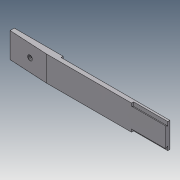
# Autodesk Inventor part: J007777 IMEC DOVE TAIL EXTENSION Rev -
Saved by Autodesk Inventor 2018.3 (Build 223284000, 284)
## iProperties
Created: 2017-01-23
Material: ALUMINUM, 6061-T651
Vendor: HHMI: JRC - ID&F
Document SubType Name: Modeling
Designer: ARNOLDJ
Density: 2.7 g/cm^3
Appearance: Metal-AL-6061 (Machined)
Description: IMEC DOVE TAIL EXTENSION
Project: COMMON
Part Number: J007777 IMEC DOVE TAIL EXTENSION Rev -
RuleStatus: InUse
AfterDocSave0: file://Part Number Cleaner
LAB/DEPT: APIG (SHARED RESOURCE)
REQUESTING SCIENTIST: BARBARTIS, BRIAN
SURFACE ROUGHNESS: 32 Ra
DESIGN DEPARTMENT: HHMI: JRC - ID&F
SPECIAL FINISH: NONE
ALTERED ITEM PART NUMBER: N/A
ALTERED ITEM VENDOR: N/A
ALTERED ITEM DESCRIPTION: N/A
Author: ARNOLDJ
Revision Number: 0
Autodesk Inventor part; units mm, degrees
ref_plane "YZ Plane" through (0, 0, 0) normal (1, 0, 0) x (0, 1, 0)
ref_plane "XZ Plane" through (0, 0, 0) normal (0, 1, 0) x (-1, 0, 0)
ref_plane "XY Plane" through (0, 0, 0) normal (0, 0, 1) x (1, 0, 0)
sketch "Sketch1" plane through (0, 0, 0) normal (0, 0, 1) x (1, 0, 0)
  line L0 (0, 4.2672) -> (0, -4.2672) projected
  line L1 (-26.67, 0) -> (26.67, 0) projected
  line L2 (19.05, -3.048) -> (-19.05, -3.048)
  line L3 (-19.05, -3.048) -> (-19.05, 3.048)
  line L4 (-19.05, 3.048) -> (19.05, 3.048)
  line L5 (19.05, 3.048) -> (19.05, -3.048)
  line L6 (19.05, -3.048) -> (-19.05, 3.048) construction
  line L7 (-19.05, -3.048) -> (19.05, 3.048) construction
  point P0 (0, 0)
  dimension "d0" = 38.1
  dimension "d1" = 6.096
  constraints: 12 end point, 2 midpoint, 2 parallel, 1 horizontal, 1 perpendicular
  measures "d0" distance of L3.end L4.end
  measures "d1" distance of L2.end L3.end
extrude "Extrusion1" add sketch "Sketch1" along normal blind 1.016
sketch "Sketch2" plane through (19.05, -3.048, 0) normal (1, 0, 0) x (0, 0, -1)
  line L0 (0, 0) -> (-1.016, 0) projected
  line L1 (-1.016, 0) -> (-1.016, 6.096) projected
  line L2 (0, 6.096) -> (0, 0) projected
  line L3 (-0.508, 0) -> (-0.508, 0.9474)
  line L4 (-0.508, 0.9474) -> (-1.016, 0.6541)
  line L5 (-1.016, 0.6541) -> (-1.016, 0)
  line L6 (-1.016, 0) -> (-0.508, 0)
  line L7 (-1.2192, 3.048) -> (0.2032, 3.048) projected
  point P0 (0, 3.048)
  dimension "d4" = 0.508
  dimension "d5" = 0.9474
  dimension "d6" = 60
  dimension "d15" = 0.6541
  dimension "d16" = 2.1006
  constraints: 8 end point, 2 perpendicular, 1 collinear, 1 midpoint, 1 point on line
  measures "d4" distance between parallel lines of L3 L1
  measures "d5" distance of L3.start L3.end
  measures "d6" angle of L3 L4
  measures "d15" distance from line of L0 L4.end
  measures "d16" distance from line of L3.end L7
extrude "Extrusion2" cut sketch "Sketch2" against normal blind 8.255 contours L0 L1 L4 L3
mirror "Mirror1" about plane through (0, 0, 0) normal (0, 1, 0) of "Extrusion2"
sketch "Sketch4" plane through (0, 0, 0) normal (0, 0, -1) x (-1, 0, 0)
  line L0 (-19.05, -3.048) -> (19.05, -3.048) projected
  line L1 (19.05, -3.048) -> (19.05, 3.048) projected
  line L2 (19.05, 3.048) -> (-19.05, 3.048) projected
  line L3 (-19.05, 3.048) -> (-19.05, -3.048) projected
  line L4 (-26.67, 0) -> (26.67, 0) projected
  line L5 (7.239, -3.048) -> (19.05, -3.048)
  line L6 (19.05, -3.048) -> (19.05, 3.048)
  line L7 (19.05, 3.048) -> (7.239, 3.048)
  line L8 (7.239, 3.048) -> (7.239, -3.048)
  line L9 (7.239, -3.048) -> (19.05, 3.048) construction
  line L10 (19.05, -3.048) -> (7.239, 3.048) construction
  point P0 (0, 0)
  point P1 (13.1445, 0)
  dimension "d17" = 11.811
  constraints: 12 end point, 2 midpoint, 2 parallel, 1 horizontal, 1 perpendicular, 1 point on line
  measures "d17" distance between parallel lines of L1 L8
extrude "Extrusion4" add sketch "Sketch4" along normal blind 0.508 contours L8 L4 L1 L0 | L8 L2 L1 L4
sketch "Sketch5" plane through (-19.05, -3.048, 1.016) normal (-1, 0, 0) x (0, 0, 1)
  line L0 (-1.8288, 3.048) -> (0.3048, 3.048) projected
  line L1 (-1.016, 7.3152) -> (-1.016, -1.2192) projected
  line L2 (-1.524, 0) -> (-1.524, 6.096) projected
  line L3 (-1.524, 6.096) -> (-1.524, 0) projected
  line L4 (-1.524, 0.9398) -> (-0.9652, 0.6172)
  line L5 (-0.9652, 0.6172) -> (-0.9652, 5.4788)
  line L6 (-0.9652, 5.4788) -> (-1.524, 5.1562)
  line L7 (-1.524, 0.9398) -> (-1.524, 5.1562)
  point P0 (-1.016, 3.048)
  dimension "d20" = 60
  dimension "d21" = 60
  dimension "d22" = 2.1082
  dimension "d23" = 4.2164
  dimension "d24" = 0.5588
  constraints: 8 end point, 2 point on line, 1 parallel, 1 vertical
  measures "d20" angle of L4 L5
  measures "d21" angle of L5 L6
  measures "d22" distance from line of L0 L6.end
  measures "d23" distance of L6.end L4.start
  measures "d24" distance between parallel lines of L5 L2
extrude "Extrusion5" cut sketch "Sketch5" against normal blind 9.652
sketch "Sketch6" plane through (-19.05, -2.4308, 0.0508) normal (0, 0, -1) x (-1, 0, 0)
  line L0 (0, 4.8616) -> (0, 0) projected
  line L1 (0, 4.8616) -> (-9.652, 4.8616) projected
  line L2 (-9.652, 4.8616) -> (-9.652, 0) projected
  line L3 (0, 0) -> (-9.652, 0) projected
  line L4 (-45.72, 2.4308) -> (7.62, 2.4308) projected
  point P0 (-19.05, 2.4308)
  point P1 (-5.08, 2.4308)
  dimension "d27" = 5.08
  constraints: 1 point on line
  measures "d27" distance from line of L0 point (-5.08, 2.431)
hole "Hole1" at (-13.97, 0, 0.0508) direction (0, 0, 1) diameter 1.1938 end through all
chamfer "Chamfer1" distance 9.271 distance2 0.508 1 edges at (-19.05, 0, 1.016) measured on face at (-18.55, 0, 1.016)
fillet "Fillet2" radius 1.016 2 edges at (-9.398, 2.2695, -0.2286) (-9.398, -2.2695, -0.2286)
equation "\"d23\" = 2 * d22"
body "Solid1"
